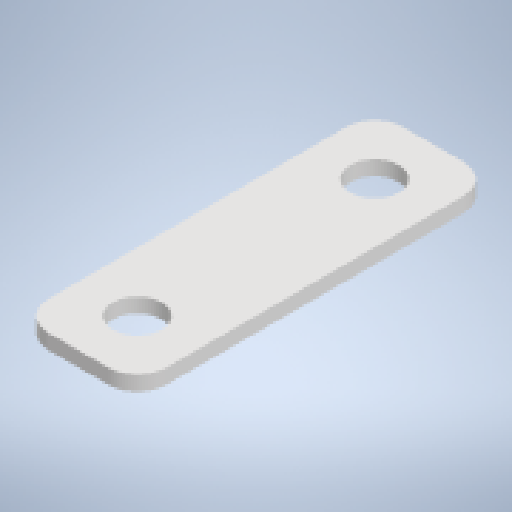
# Autodesk Inventor part: Triangle spacer
Saved by Autodesk Inventor 2023 (Build 270158000, 158)
## iProperties
Created: 2023-03-06
Part Number: Triangle spacer
Material: Generic
Document SubType Name: Modeling
Designer: Gabriel - T3 CAD
Density: 1 g/cm^3
Appearance: Default
Author: Gabriel - T3 CAD
Autodesk Inventor part; units mm, degrees
ref_plane "YZ Plane" through (0, 0, 0) normal (1, 0, 0) x (0, 1, 0)
ref_plane "XZ Plane" through (0, 0, 0) normal (0, 1, 0) x (-1, 0, 0)
ref_plane "XY Plane" through (0, 0, 0) normal (0, 0, 1) x (1, 0, 0)
sketch "Sketch1" plane through (0, 0, 0) normal (0, 1, 0) x (-1, 0, 0)
  line L0 (3.175, 0) -> (9.525, 0)
  line L1 (12.7, 3.175) -> (12.7, 34.925)
  line L2 (9.525, 38.1) -> (3.175, 38.1)
  line L3 (0, 34.925) -> (0, 3.175)
  arc A0 (12.7, 34.925) -> (9.525, 38.1) centre (9.525, 34.925) ccw
  arc A1 (3.175, 38.1) -> (0, 34.925) centre (3.175, 34.925) ccw
  arc A2 (0, 3.175) -> (3.175, 0) centre (3.175, 3.175) ccw
  arc A3 (9.525, 0) -> (12.7, 3.175) centre (9.525, 3.175) ccw
  circle A4 centre (6.35, 31.75) radius 2.5797
  circle A5 centre (6.35, 6.35) radius 2.5797
  point P0 (0, 0)
  point P1 (12.7, 38.1)
  point P2 (12.7, 0)
  point P3 (0, 38.1)
  dimension "d0" = 12.7
  dimension "d1" = 38.1
  dimension "d2" = 3.175
  dimension "d3" = 25.4
  dimension "d4" = 6.35
  dimension "d5" = 6.35
  dimension "d6" = 6.35
  dimension "d7" = 5.1594
  constraints: 8 end point, 8 point on circle, 8 point on line, 8 tangent, 6 centre point, 4 equal radius, 2 parallel, 1 horizontal, 1 perpendicular
  measures "d0" distance of point (0, 38.1) point (12.7, 38.1)
  measures "d1" distance of point (12.7, 38.1) point (12.7, 0)
  measures "d2" radius of A0
  measures "d3" distance of A4.centre A5.centre
  measures "d4" distance from line of L0 A5.centre
  measures "d5" distance from line of L3 A5.centre
  measures "d6" distance from line of L3 A4.centre
  measures "d7" diameter of A5
extrude "Extrusion1" add sketch "Sketch1" along normal blind 1.5875
equation "\"d5\" = d4"
equation "\"d6\" = d5"
body "Solid1"
